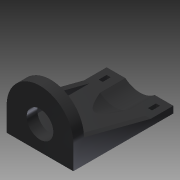
# Autodesk Inventor part: proxxon_mount
Saved by Autodesk Inventor 2013 (Build 170138000, 138)
## iProperties
Created: 2014-01-31
Part Number: proxxon_mount
Material: Generic
Document SubType Name: Modeling
Designer: Masta
Density: 1 g/cm^3
Author: Masta
Autodesk Inventor part; units mm, degrees
ref_plane "YZ Plane" through (0, 0, 0) normal (1, 0, 0) x (0, 1, 0)
ref_plane "XZ Plane" through (0, 0, 0) normal (0, 1, 0) x (-1, 0, 0)
ref_plane "XY Plane" through (0, 0, 0) normal (0, 0, 1) x (1, 0, 0)
sketch "Sketch1" plane through (0, 0, 0) normal (0, 0, 1) x (1, 0, 0)
  line L0 (-25, -25) -> (25, -25)
  line L1 (25, -25) -> (25, 25)
  line L2 (25, 25) -> (-25, 25)
  line L3 (-25, 25) -> (-25, -25)
  line L4 (-25, -25) -> (25, 25) construction
  line L5 (25, -25) -> (-25, 25) construction
  line L6 (-25, 0) -> (25, 0) construction
  circle A0 centre (-12, 0) radius 1.75
  line L7 (0, 25) -> (0, -25) construction
  circle A1 centre (12, 0) radius 1.75
  line L8 (-25, 25) -> (25, 25)
  line L9 (25, 25) -> (25, 50)
  line L10 (25, 50) -> (-25, 50)
  line L11 (-25, 50) -> (-25, 25)
  line L12 (-20, 45) -> (-17, 45)
  line L13 (-17, 45) -> (-17, 39)
  line L14 (-17, 39) -> (-20, 39)
  line L15 (-20, 39) -> (-20, 45)
  line L16 (20, 45) -> (17, 45)
  line L17 (17, 45) -> (17, 39)
  line L18 (17, 39) -> (20, 39)
  line L19 (20, 39) -> (20, 45)
  point P0 (0, 0)
  dimension "d0" = 50
  dimension "d1" = 50
  dimension "d14" = 3.5
  dimension "d15" = 24
  dimension "d16" = 25
  dimension "d17" = 5
  dimension "d18" = 6
  dimension "d19" = 3
  dimension "d20" = 17
  constraints: 40 end point, 6 midpoint, 6 parallel, 5 symmetric about line, 3 horizontal, 3 perpendicular, 2 centre point, 2 collinear, 2 point on line, 1 other
  measures "d0" distance of L2.end L1.end
  measures "d1" distance of L1.end L0.end
  measures "d14" diameter of A0
  measures "d15" distance of A1.centre A0.centre
  measures "d16" distance of L9.end L8.end
  measures "d17" distance between parallel lines of L10 L12
  measures "d18" distance of L14.end L12.start
  measures "d19" distance of L13.end L14.end
  measures "d20" distance between parallel lines of L13 L7
extrude "Extrusion1" add sketch "Sketch1" along normal blind 5
sketch "Sketch2" plane through (-25, -25, 0) normal (0, -1, 0) x (1, 0, 0)
  line L0 (0, 0) -> (50, 0) projected
  line L1 (0, 5) -> (50, 5) projected
  line L2 (0, 0) -> (0, 5) projected
  circle A0 centre (25, 18) radius 10
  circle A1 centre (25, 18) radius 17 construction
  line L3 (25, 18) -> (25, 0) construction
  line L4 (0, 5) -> (0, 18)
  arc A2 (50, 18) -> (0, 18) centre (25, 18) ccw
  line L5 (50, 18) -> (50, 5)
  dimension "d4" = 20
  dimension "d5" = 34
  dimension "d6" = 18
  constraints: 6 end point, 3 centre point, 3 parallel, 2 coincident, 2 point on circle, 2 tangent
  measures "d4" diameter of A0
  measures "d5" diameter of A1
  measures "d6" distance from line of L0 L3.start
extrude "Extrusion2" add sketch "Sketch2" against normal blind 8
sketch "Sketch3" plane through (0, 0, 0) normal (1, 0, 0) x (0, 1, 0)
  line L0 (-17, 28) -> (-25, 28) projected
  line L1 (-17, 8) -> (-17, 5) projected
  line L2 (-17, 5) -> (50, 5) projected
  line L3 (50, 0) -> (-25, 0) projected
  line L4 (-25, 0) -> (-25, 8) projected
  line L5 (-25, 43) -> (-17, 43) projected
  line L6 (-17, 43) -> (-17, 28) projected
  line L7 (-25, 8) -> (-17, 8) projected
  line L8 (-25, 28) -> (-25, 43) projected
  line L9 (-25, 8) -> (-25, 28)
  line L10 (-25, 18) -> (31, 18)
  line L11 (9, 29) -> (31, 35)
  line L12 (31, 18) -> (31, 35)
  line L13 (50, 5) -> (50, 0) projected
  line L14 (9, 29) -> (-17, 28)
  line L15 (31, 18) -> (56.5287, 18)
  line L16 (56.5287, 18) -> (56.5287, 35)
  line L17 (56.5287, 35) -> (31, 35)
  line L18 (31, 35) -> (31, 18)
  point P0 (0, 0)
  dimension "d9" = 26
  dimension "d10" = 22
  dimension "d11" = 11
  dimension "d12" = 17
  constraints: 18 end point, 3 perpendicular, 2 parallel, 1 collinear, 1 horizontal, 1 midpoint
  measures "d9" horizontal distance of L1.start L11.start
  measures "d10" horizontal distance of L11.start L11.end
  measures "d11" distance from line of L10 L11.start
  measures "d12" distance from line of L11.end L10
revolve "Revolution1" cut sketch "Sketch3" angle 360 about axis through (0, -25, 18) along (0, 1, 0) contours L14 L11 L12 L10 L9 L0 | L17 L16 L15 L12
sketch "Sketch4" plane through (-25, -25, 0) normal (-1, 0, 0) x (0, 0, 1)
  line L0 (5, 8) -> (18, 8) projected
  line L1 (5, 75) -> (5, 8) projected
  line L2 (18, 8) -> (5, 58)
  point P0 (0, 25)
  dimension "d21" = 50
  constraints: 2 end point, 1 point on line
  measures "d21" distance from line of L0 L2.end
extrude "Extrusion3" add sketch "Sketch4" against normal blind 4
mirror "Mirror1" about plane through (0, 0, 0) normal (1, 0, 0) of "Extrusion3"
body "Solid1"
